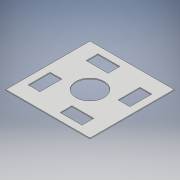
# Autodesk Inventor part: Peça5
Saved by Autodesk Inventor 2018 (Build 220112000, 112)
## iProperties
Created: 2018-05-04
Part Number: Peça5
Material: Genérico
Document SubType Name: Chapa de metal
Designer: Georgines
Density: 1 g/cm^3
Appearance: Padrão
Sheet Metal Rule: Padrão_mm
Author: Georgines
Autodesk Inventor part; units mm, degrees
ref_plane "YZ Plane" through (0, 0, 0) normal (1, 0, 0) x (0, 1, 0)
ref_plane "XZ Plane" through (0, 0, 0) normal (0, 1, 0) x (-1, 0, 0)
ref_plane "XY Plane" through (0, 0, 0) normal (0, 0, 1) x (1, 0, 0)
sketch "Esboço1" plane through (0, 0, 0) normal (0, 0, 1) x (1, 0, 0)
  line L0 (62, -26) -> (-138, -26) construction
  line L1 (-121, 5) -> (-93, 5)
  line L2 (-93, 5) -> (-93, 57)
  line L3 (-93, 57) -> (-121, 57)
  line L4 (-121, 57) -> (-121, 5)
  line L5 (-121, 5) -> (-93, 57) construction
  line L6 (-93, 5) -> (-121, 57) construction
  line L7 (-102, 124) -> (-50, 124)
  line L8 (-50, 124) -> (-50, 152)
  line L9 (-50, 152) -> (-102, 152)
  line L10 (-102, 152) -> (-102, 124)
  line L11 (-102, 124) -> (-50, 152) construction
  line L12 (-50, 124) -> (-102, 152) construction
  line L13 (-26, -14) -> (26, -14)
  line L14 (26, -14) -> (26, 14)
  line L15 (26, 14) -> (-26, 14)
  line L16 (-26, 14) -> (-26, -14)
  line L17 (-26, -14) -> (26, 14) construction
  line L18 (26, -14) -> (-26, 14) construction
  line L19 (17, 81) -> (45, 81)
  line L20 (45, 81) -> (45, 133)
  line L21 (45, 133) -> (17, 133)
  line L22 (17, 133) -> (17, 81)
  line L23 (17, 81) -> (45, 133) construction
  line L24 (45, 81) -> (17, 133) construction
  line L25 (-138, 134.0702) -> (-38, 134.0702) construction
  line L26 (-38, 134.0702) -> (-38, -26) construction
  line L27 (-38, 134.0702) -> (62, 134.0702) construction
  line L28 (-38, 169) -> (-38, 69) construction
  circle A0 centre (-38, 69) radius 33.5
  line L29 (-138, 169) -> (62, 169)
  line L30 (62, 169) -> (62, -31)
  line L31 (62, -31) -> (-138, -31)
  line L32 (-138, -31) -> (-138, 169)
  line L33 (-138, 169) -> (62, -31) construction
  line L34 (62, 169) -> (-138, -31) construction
  point P0 (0, 0)
  point P1 (-107, 31)
  point P2 (-76, 138)
  point P3 (31, 107)
  dimension "d0" = 28
  dimension "d1" = 52
  dimension "d2" = 52
  dimension "d3" = 28
  dimension "d4" = 52
  dimension "d5" = 28
  dimension "d6" = 28
  dimension "d7" = 52
  dimension "d8" = 100
  dimension "d9" = 100
  dimension "d10" = 67
  dimension "d11" = 200
  dimension "d12" = 200
  constraints: 70 end point, 11 midpoint, 10 parallel, 6 horizontal, 5 perpendicular, 3 point on line, 1 centre point, 1 coincident
  measures "d0" distance of L3.end L2.end
  measures "d1" distance of L2.end L1.end
  measures "d2" distance of L9.end L8.end
  measures "d3" distance of L8.end L7.end
  measures "d4" distance of L15.end L14.end
  measures "d5" distance of L14.end L13.end
  measures "d6" distance of L21.end L20.end
  measures "d7" distance of L20.end L19.end
  measures "d8" distance of L25.start L25.end
  measures "d9" distance of L28.start L28.end
  measures "d10" diameter of A0
  measures "d11" distance of L30.end L31.end
  measures "d12" distance of L29.end L30.end
extrude "Extrusão1" add sketch "Esboço1" along normal blind 2
equation "\"Raio_vergadura\" = Espessura"
equation "\"Largura_alívio_de_vergadura\" = Espessura"
equation "\"Profundidade_alívio_de_vergadura\" = 0.5 * Espessura"
equation "\"Tamanho_alívio_de_dobra\" = 4 * Espessura"
equation "\"Remanescente_mínimo\" = 2 * Espessura"
equation "\"Raiodetransição\" = Raio_vergadura"
equation "\"Tamanho_de_raio_de_Jacobi\" = Raio_vergadura"
equation "\"TamanhoFolga\" = Espessura"
equation "\"Espessura\" = 2"
